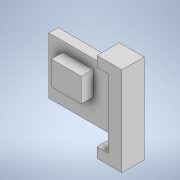
# Autodesk Inventor part: heatsink_2
Saved by Autodesk Inventor 2021 (Build 250183000, 183)
## iProperties
Created: 2021-09-27
Part Number: heatsink_2
Material: Generic
Document SubType Name: Modeling
Designer: Administrator
Density: 1 g/cm^3
Appearance: Default
Author: Administrator
Autodesk Inventor part; units mm, degrees
ref_plane "YZ Plane" through (0, 0, 0) normal (1, 0, 0) x (0, 1, 0)
ref_plane "XZ Plane" through (0, 0, 0) normal (0, 1, 0) x (-1, 0, 0)
ref_plane "XY Plane" through (0, 0, 0) normal (0, 0, 1) x (1, 0, 0)
sketch "Sketch8" plane through (0, 0, 0) normal (0, 0, 1) x (1, 0, 0)
  line L0 (-23.4899, -4.07) -> (-4.7399, -4.07)
  line L1 (-4.7399, -4.07) -> (-4.7399, 10.93)
  line L2 (-4.7399, 10.93) -> (-23.4899, 10.93)
  line L3 (-23.4899, 10.93) -> (-23.4899, -4.07)
  line L4 (5.9, -21.53) -> (12.9, -21.53)
  line L5 (12.9, -21.53) -> (12.9, 21.53)
  line L6 (12.9, 21.53) -> (5.9, 21.53)
  line L7 (9.6, -27.93) -> (13.2, -27.93)
  line L8 (-21.4963, 16.93) -> (5.9, 16.93)
  line L9 (5.9, 16.93) -> (5.9, 27.93)
  line L10 (5.9, 27.93) -> (21.5, 27.93)
  line L11 (21.5, 27.93) -> (21.5, -27.93)
  line L12 (21.5, -27.93) -> (5.9, -27.93)
  line L13 (5.9, -27.93) -> (5.9, -18.57)
  line L14 (5.9, -18.57) -> (-21.4789, -18.57)
  line L15 (-21.4789, -18.57) -> (-32.4963, -18.57)
  line L16 (-32.4963, -18.57) -> (-32.4963, 16.93)
  line L17 (-32.4963, 16.93) -> (-21.4963, 16.93)
  point P0 (0, 0)
  point P1 (5.9, -27.93)
  constraints: 36 end point
extrude "Extrusion10" add sketch "Sketch8" along normal blind 14 contours L4 L5 L6 L9 L10 L11 L12 L7 L13
extrude "Extrusion11" add sketch "Sketch8" along normal blind 13.2 contours L3 L2 L1 L0
extrude "Extrusion12" add sketch "Sketch8" along normal blind 5.8 contours L13 L14 L15 L16 L17 L8 L9 L6 L5 L4
body "Solid4"
